抽篮子 (Autodesk Fusion 360 design; units mm, degrees)
part number: 2026-05-02-11-19-45-194
Autodesk Fusion 360 part; units mm, degrees
(part 1 of 4)
sketch "草图1" plane through (0, 0, 0) normal (0, 0, 1) x (1, 0, 0)
  line L0 (-125, -56.5) -> (125, -56.5)
  line L1 (125, -56.5) -> (125, 56.5)
  line L2 (125, 56.5) -> (-125, 56.5)
  line L3 (-125, 56.5) -> (-125, -56.5)
  point P0 (0, -56.5)
  point P1 (-125, 0)
  dimension "d13" = 250
  dimension "d14" = 113
  constraint horizontal L0
  constraint horizontal L2
  constraint vertical L3
  constraint vertical L1
  constraint midpoint L0 P0
  constraint midpoint L3 P1
  constraint vertical origin P0
  constraint horizontal origin P1
  measures "d13" horizontal distance of L0.start L0.end
  measures "d14" vertical distance of L0.start L2.end
extrude "拉伸1" add sketch "草图1" along normal blind 90
fillet "fillet_right_corners" radius 10 2 edges at (125, 56.5, 45) (125, -56.5, 45)
shell "shell_basket" thickness 2 removed faces 1 at (-45, 18.8333, 90)
sketch "草图16" plane through (125, 0, 0) normal (1, 0, 0) x (0, 1, 0)
  line L0 (-46.5, 90) -> (-46.5, 0)
  line L1 (-46.5, 0) -> (46.5, 0)
  line L2 (46.5, 0) -> (46.5, 90)
  line L3 (46.5, 90) -> (-46.5, 90)
  arc A0 (29, 60) -> (29, 82) centre (29, 71) ccw
  arc A1 (-29, 82) -> (-29, 60) centre (-29, 71) ccw
  line L4 (-29, 60) -> (29, 60)
  line L5 (29, 82) -> (-29, 82)
  dimension "d60" = 29
  dimension "d61" = 29
  dimension "d62" = 71
  dimension "d63" = 11
  dimension "d64" = 11
  constraint horizontal L4
  constraint horizontal L5
  constraint horizontal A0.centre A1.centre
  measures "d60" horizontal distance of origin A1.centre
  measures "d61" horizontal distance of origin A0.centre
  measures "d62" vertical distance of origin A1.centre
  measures "d63" radius of A1
  measures "d64" radius of A0
extrude "拉伸16" cut sketch "草图16" against normal blind 3 contours A0 A1 L4 L5
sketch "草图29" plane through (-125, 0, 0) normal (-1, 0, 0) x (0, -1, 0)
  line L0 (-56.5, 0) -> (56.5, 0)
  line L1 (56.5, 0) -> (56.5, 90)
  line L2 (56.5, 90) -> (-56.5, 90)
  line L3 (-56.5, 90) -> (-56.5, 0)
  line L4 (-47.5, 14) -> (-51.8301, 11.5)
  line L5 (-51.8301, 11.5) -> (-51.8301, 6.5)
  line L6 (-51.8301, 6.5) -> (-47.5, 4)
  line L7 (-47.5, 4) -> (-43.1699, 6.5)
  line L8 (-43.1699, 6.5) -> (-43.1699, 11.5)
  line L9 (-43.1699, 11.5) -> (-47.5, 14)
  line L10 (-36.8397, 14) -> (-41.1699, 11.5)
  line L11 (-41.1699, 11.5) -> (-41.1699, 6.5)
  line L12 (-41.1699, 6.5) -> (-36.8397, 4)
  line L13 (-36.8397, 4) -> (-32.5096, 6.5)
  line L14 (-32.5096, 6.5) -> (-32.5096, 11.5)
  line L15 (-32.5096, 11.5) -> (-36.8397, 14)
  line L16 (-26.1795, 14) -> (-30.5096, 11.5)
  line L17 (-30.5096, 11.5) -> (-30.5096, 6.5)
  line L18 (-30.5096, 6.5) -> (-26.1795, 4)
  line L19 (-26.1795, 4) -> (-21.8494, 6.5)
  line L20 (-21.8494, 6.5) -> (-21.8494, 11.5)
  line L21 (-21.8494, 11.5) -> (-26.1795, 14)
  line L22 (-15.5192, 14) -> (-19.8494, 11.5)
  line L23 (-19.8494, 11.5) -> (-19.8494, 6.5)
  line L24 (-19.8494, 6.5) -> (-15.5192, 4)
  line L25 (-15.5192, 4) -> (-11.1891, 6.5)
  line L26 (-11.1891, 6.5) -> (-11.1891, 11.5)
  line L27 (-11.1891, 11.5) -> (-15.5192, 14)
  line L28 (-4.859, 14) -> (-9.1891, 11.5)
  line L29 (-9.1891, 11.5) -> (-9.1891, 6.5)
  line L30 (-9.1891, 6.5) -> (-4.859, 4)
  line L31 (-4.859, 4) -> (-0.5289, 6.5)
  line L32 (-0.5289, 6.5) -> (-0.5289, 11.5)
  line L33 (-0.5289, 11.5) -> (-4.859, 14)
  line L34 (5.8013, 14) -> (1.4711, 11.5)
  line L35 (1.4711, 11.5) -> (1.4711, 6.5)
  line L36 (1.4711, 6.5) -> (5.8013, 4)
  line L37 (5.8013, 4) -> (10.1314, 6.5)
  line L38 (10.1314, 6.5) -> (10.1314, 11.5)
  line L39 (10.1314, 11.5) -> (5.8013, 14)
  line L40 (16.4615, 14) -> (12.1314, 11.5)
  line L41 (12.1314, 11.5) -> (12.1314, 6.5)
  line L42 (12.1314, 6.5) -> (16.4615, 4)
  line L43 (16.4615, 4) -> (20.7917, 6.5)
  line L44 (20.7917, 6.5) -> (20.7917, 11.5)
  line L45 (20.7917, 11.5) -> (16.4615, 14)
  line L46 (27.1218, 14) -> (22.7917, 11.5)
  line L47 (22.7917, 11.5) -> (22.7917, 6.5)
  line L48 (22.7917, 6.5) -> (27.1218, 4)
  line L49 (27.1218, 4) -> (31.4519, 6.5)
  line L50 (31.4519, 6.5) -> (31.4519, 11.5)
  line L51 (31.4519, 11.5) -> (27.1218, 14)
  line L52 (37.782, 14) -> (33.4519, 11.5)
  line L53 (33.4519, 11.5) -> (33.4519, 6.5)
  line L54 (33.4519, 6.5) -> (37.782, 4)
  line L55 (37.782, 4) -> (42.1122, 6.5)
  line L56 (42.1122, 6.5) -> (42.1122, 11.5)
  line L57 (42.1122, 11.5) -> (37.782, 14)
  line L58 (-42.1699, 23.2321) -> (-46.5, 20.7321)
  line L59 (-46.5, 20.7321) -> (-46.5, 15.7321)
  line L60 (-46.5, 15.7321) -> (-42.1699, 13.2321)
  line L61 (-42.1699, 13.2321) -> (-37.8397, 15.7321)
  line L62 (-37.8397, 15.7321) -> (-37.8397, 20.7321)
  line L63 (-37.8397, 20.7321) -> (-42.1699, 23.2321)
  line L64 (-31.5096, 23.2321) -> (-35.8397, 20.7321)
  line L65 (-35.8397, 20.7321) -> (-35.8397, 15.7321)
  line L66 (-35.8397, 15.7321) -> (-31.5096, 13.2321)
  line L67 (-31.5096, 13.2321) -> (-27.1795, 15.7321)
  line L68 (-27.1795, 15.7321) -> (-27.1795, 20.7321)
  line L69 (-27.1795, 20.7321) -> (-31.5096, 23.2321)
  line L70 (-20.8494, 23.2321) -> (-25.1795, 20.7321)
  line L71 (-25.1795, 20.7321) -> (-25.1795, 15.7321)
  line L72 (-25.1795, 15.7321) -> (-20.8494, 13.2321)
  line L73 (-20.8494, 13.2321) -> (-16.5192, 15.7321)
  line L74 (-16.5192, 15.7321) -> (-16.5192, 20.7321)
  line L75 (-16.5192, 20.7321) -> (-20.8494, 23.2321)
  line L76 (-10.1891, 23.2321) -> (-14.5192, 20.7321)
  line L77 (-14.5192, 20.7321) -> (-14.5192, 15.7321)
  line L78 (-14.5192, 15.7321) -> (-10.1891, 13.2321)
  line L79 (-10.1891, 13.2321) -> (-5.859, 15.7321)
  line L80 (-5.859, 15.7321) -> (-5.859, 20.7321)
  line L81 (-5.859, 20.7321) -> (-10.1891, 23.2321)
  line L82 (0.4711, 23.2321) -> (-3.859, 20.7321)
  line L83 (-3.859, 20.7321) -> (-3.859, 15.7321)
  line L84 (-3.859, 15.7321) -> (0.4711, 13.2321)
  line L85 (0.4711, 13.2321) -> (4.8013, 15.7321)
  line L86 (4.8013, 15.7321) -> (4.8013, 20.7321)
  line L87 (4.8013, 20.7321) -> (0.4711, 23.2321)
  line L88 (11.1314, 23.2321) -> (6.8013, 20.7321)
  line L89 (6.8013, 20.7321) -> (6.8013, 15.7321)
  line L90 (6.8013, 15.7321) -> (11.1314, 13.2321)
  line L91 (11.1314, 13.2321) -> (15.4615, 15.7321)
  line L92 (15.4615, 15.7321) -> (15.4615, 20.7321)
  line L93 (15.4615, 20.7321) -> (11.1314, 23.2321)
  line L94 (21.7917, 23.2321) -> (17.4615, 20.7321)
  line L95 (17.4615, 20.7321) -> (17.4615, 15.7321)
  line L96 (17.4615, 15.7321) -> (21.7917, 13.2321)
  line L97 (21.7917, 13.2321) -> (26.1218, 15.7321)
  line L98 (26.1218, 15.7321) -> (26.1218, 20.7321)
  line L99 (26.1218, 20.7321) -> (21.7917, 23.2321)
  line L100 (32.4519, 23.2321) -> (28.1218, 20.7321)
  line L101 (28.1218, 20.7321) -> (28.1218, 15.7321)
  line L102 (28.1218, 15.7321) -> (32.4519, 13.2321)
  line L103 (32.4519, 13.2321) -> (36.782, 15.7321)
  line L104 (36.782, 15.7321) -> (36.782, 20.7321)
  line L105 (36.782, 20.7321) -> (32.4519, 23.2321)
  line L106 (43.1122, 23.2321) -> (38.782, 20.7321)
  line L107 (38.782, 20.7321) -> (38.782, 15.7321)
  line L108 (38.782, 15.7321) -> (43.1122, 13.2321)
  line L109 (43.1122, 13.2321) -> (47.4423, 15.7321)
  line L110 (47.4423, 15.7321) -> (47.4423, 20.7321)
  line L111 (47.4423, 20.7321) -> (43.1122, 23.2321)
  line L112 (-47.5, 32.4641) -> (-51.8301, 29.9641)
  line L113 (-51.8301, 29.9641) -> (-51.8301, 24.9641)
  line L114 (-51.8301, 24.9641) -> (-47.5, 22.4641)
  line L115 (-47.5, 22.4641) -> (-43.1699, 24.9641)
  line L116 (-43.1699, 24.9641) -> (-43.1699, 29.9641)
  line L117 (-43.1699, 29.9641) -> (-47.5, 32.4641)
  line L118 (-36.8397, 32.4641) -> (-41.1699, 29.9641)
  line L119 (-41.1699, 29.9641) -> (-41.1699, 24.9641)
  line L120 (-41.1699, 24.9641) -> (-36.8397, 22.4641)
  line L121 (-36.8397, 22.4641) -> (-32.5096, 24.9641)
  line L122 (-32.5096, 24.9641) -> (-32.5096, 29.9641)
  line L123 (-32.5096, 29.9641) -> (-36.8397, 32.4641)
  line L124 (-26.1795, 32.4641) -> (-30.5096, 29.9641)
  line L125 (-30.5096, 29.9641) -> (-30.5096, 24.9641)
  line L126 (-30.5096, 24.9641) -> (-26.1795, 22.4641)
  line L127 (-26.1795, 22.4641) -> (-21.8494, 24.9641)
  line L128 (-21.8494, 24.9641) -> (-21.8494, 29.9641)
  line L129 (-21.8494, 29.9641) -> (-26.1795, 32.4641)
  line L130 (-15.5192, 32.4641) -> (-19.8494, 29.9641)
  line L131 (-19.8494, 29.9641) -> (-19.8494, 24.9641)
  line L132 (-19.8494, 24.9641) -> (-15.5192, 22.4641)
  line L133 (-15.5192, 22.4641) -> (-11.1891, 24.9641)
  line L134 (-11.1891, 24.9641) -> (-11.1891, 29.9641)
  line L135 (-11.1891, 29.9641) -> (-15.5192, 32.4641)
  line L136 (-4.859, 32.4641) -> (-9.1891, 29.9641)
  line L137 (-9.1891, 29.9641) -> (-9.1891, 24.9641)
  line L138 (-9.1891, 24.9641) -> (-4.859, 22.4641)
  line L139 (-4.859, 22.4641) -> (-0.5289, 24.9641)
  line L140 (-0.5289, 24.9641) -> (-0.5289, 29.9641)
  line L141 (-0.5289, 29.9641) -> (-4.859, 32.4641)
  line L142 (5.8013, 32.4641) -> (1.4711, 29.9641)
  line L143 (1.4711, 29.9641) -> (1.4711, 24.9641)
  line L144 (1.4711, 24.9641) -> (5.8013, 22.4641)
  line L145 (5.8013, 22.4641) -> (10.1314, 24.9641)
  line L146 (10.1314, 24.9641) -> (10.1314, 29.9641)
  line L147 (10.1314, 29.9641) -> (5.8013, 32.4641)
  line L148 (16.4615, 32.4641) -> (12.1314, 29.9641)
  line L149 (12.1314, 29.9641) -> (12.1314, 24.9641)
  line L150 (12.1314, 24.9641) -> (16.4615, 22.4641)
  line L151 (16.4615, 22.4641) -> (20.7917, 24.9641)
  line L152 (20.7917, 24.9641) -> (20.7917, 29.9641)
  line L153 (20.7917, 29.9641) -> (16.4615, 32.4641)
  line L154 (27.1218, 32.4641) -> (22.7917, 29.9641)
  line L155 (22.7917, 29.9641) -> (22.7917, 24.9641)
  line L156 (22.7917, 24.9641) -> (27.1218, 22.4641)
  line L157 (27.1218, 22.4641) -> (31.4519, 24.9641)
  line L158 (31.4519, 24.9641) -> (31.4519, 29.9641)
  line L159 (31.4519, 29.9641) -> (27.1218, 32.4641)
  line L160 (37.782, 32.4641) -> (33.4519, 29.9641)
  line L161 (33.4519, 29.9641) -> (33.4519, 24.9641)
  line L162 (33.4519, 24.9641) -> (37.782, 22.4641)
  line L163 (37.782, 22.4641) -> (42.1122, 24.9641)
  line L164 (42.1122, 24.9641) -> (42.1122, 29.9641)
  line L165 (42.1122, 29.9641) -> (37.782, 32.4641)
  line L166 (-42.1699, 41.6962) -> (-46.5, 39.1962)
  line L167 (-46.5, 39.1962) -> (-46.5, 34.1962)
  line L168 (-46.5, 34.1962) -> (-42.1699, 31.6962)
  line L169 (-42.1699, 31.6962) -> (-37.8397, 34.1962)
  line L170 (-37.8397, 34.1962) -> (-37.8397, 39.1962)
  line L171 (-37.8397, 39.1962) -> (-42.1699, 41.6962)
  line L172 (-31.5096, 41.6962) -> (-35.8397, 39.1962)
  line L173 (-35.8397, 39.1962) -> (-35.8397, 34.1962)
  line L174 (-35.8397, 34.1962) -> (-31.5096, 31.6962)
  line L175 (-31.5096, 31.6962) -> (-27.1795, 34.1962)
  line L176 (-27.1795, 34.1962) -> (-27.1795, 39.1962)
  line L177 (-27.1795, 39.1962) -> (-31.5096, 41.6962)
  line L178 (-20.8494, 41.6962) -> (-25.1795, 39.1962)
  line L179 (-25.1795, 39.1962) -> (-25.1795, 34.1962)
  line L180 (-25.1795, 34.1962) -> (-20.8494, 31.6962)
  line L181 (-20.8494, 31.6962) -> (-16.5192, 34.1962)
  line L182 (-16.5192, 34.1962) -> (-16.5192, 39.1962)
  line L183 (-16.5192, 39.1962) -> (-20.8494, 41.6962)
  line L184 (-10.1891, 41.6962) -> (-14.5192, 39.1962)
  line L185 (-14.5192, 39.1962) -> (-14.5192, 34.1962)
  line L186 (-14.5192, 34.1962) -> (-10.1891, 31.6962)
  line L187 (-10.1891, 31.6962) -> (-5.859, 34.1962)
  line L188 (-5.859, 34.1962) -> (-5.859, 39.1962)
  line L189 (-5.859, 39.1962) -> (-10.1891, 41.6962)
  line L190 (0.4711, 41.6962) -> (-3.859, 39.1962)
  line L191 (-3.859, 39.1962) -> (-3.859, 34.1962)
  line L192 (-3.859, 34.1962) -> (0.4711, 31.6962)
  line L193 (0.4711, 31.6962) -> (4.8013, 34.1962)
  line L194 (4.8013, 34.1962) -> (4.8013, 39.1962)
  line L195 (4.8013, 39.1962) -> (0.4711, 41.6962)
  line L196 (11.1314, 41.6962) -> (6.8013, 39.1962)
  line L197 (6.8013, 39.1962) -> (6.8013, 34.1962)
  line L198 (6.8013, 34.1962) -> (11.1314, 31.6962)
  line L199 (11.1314, 31.6962) -> (15.4615, 34.1962)
  line L200 (15.4615, 34.1962) -> (15.4615, 39.1962)
  line L201 (15.4615, 39.1962) -> (11.1314, 41.6962)
  line L202 (21.7917, 41.6962) -> (17.4615, 39.1962)
  line L203 (17.4615, 39.1962) -> (17.4615, 34.1962)
  line L204 (17.4615, 34.1962) -> (21.7917, 31.6962)
  line L205 (21.7917, 31.6962) -> (26.1218, 34.1962)
  line L206 (26.1218, 34.1962) -> (26.1218, 39.1962)
  line L207 (26.1218, 39.1962) -> (21.7917, 41.6962)
  line L208 (32.4519, 41.6962) -> (28.1218, 39.1962)
  line L209 (28.1218, 39.1962) -> (28.1218, 34.1962)
  line L210 (28.1218, 34.1962) -> (32.4519, 31.6962)
  line L211 (32.4519, 31.6962) -> (36.782, 34.1962)
  line L212 (36.782, 34.1962) -> (36.782, 39.1962)
  line L213 (36.782, 39.1962) -> (32.4519, 41.6962)
  line L214 (43.1122, 41.6962) -> (38.782, 39.1962)
  line L215 (38.782, 39.1962) -> (38.782, 34.1962)
  line L216 (38.782, 34.1962) -> (43.1122, 31.6962)
  line L217 (43.1122, 31.6962) -> (47.4423, 34.1962)
  line L218 (47.4423, 34.1962) -> (47.4423, 39.1962)
  line L219 (47.4423, 39.1962) -> (43.1122, 41.6962)
  line L220 (-47.5, 50.9282) -> (-51.8301, 48.4282)
  line L221 (-51.8301, 48.4282) -> (-51.8301, 43.4282)
  line L222 (-51.8301, 43.4282) -> (-47.5, 40.9282)
  line L223 (-47.5, 40.9282) -> (-43.1699, 43.4282)
  line L224 (-43.1699, 43.4282) -> (-43.1699, 48.4282)
  line L225 (-43.1699, 48.4282) -> (-47.5, 50.9282)
  line L226 (-36.8397, 50.9282) -> (-41.1699, 48.4282)
  line L227 (-41.1699, 48.4282) -> (-41.1699, 43.4282)
  line L228 (-41.1699, 43.4282) -> (-36.8397, 40.9282)
  line L229 (-36.8397, 40.9282) -> (-32.5096, 43.4282)
  line L230 (-32.5096, 43.4282) -> (-32.5096, 48.4282)
  line L231 (-32.5096, 48.4282) -> (-36.8397, 50.9282)
  line L232 (-26.1795, 50.9282) -> (-30.5096, 48.4282)
  line L233 (-30.5096, 48.4282) -> (-30.5096, 43.4282)
  line L234 (-30.5096, 43.4282) -> (-26.1795, 40.9282)
  line L235 (-26.1795, 40.9282) -> (-21.8494, 43.4282)
  line L236 (-21.8494, 43.4282) -> (-21.8494, 48.4282)
  line L237 (-21.8494, 48.4282) -> (-26.1795, 50.9282)
  line L238 (-15.5192, 50.9282) -> (-19.8494, 48.4282)
  line L239 (-19.8494, 48.4282) -> (-19.8494, 43.4282)
  line L240 (-19.8494, 43.4282) -> (-15.5192, 40.9282)
  line L241 (-15.5192, 40.9282) -> (-11.1891, 43.4282)
  line L242 (-11.1891, 43.4282) -> (-11.1891, 48.4282)
  line L243 (-11.1891, 48.4282) -> (-15.5192, 50.9282)
  line L244 (-4.859, 50.9282) -> (-9.1891, 48.4282)
  line L245 (-9.1891, 48.4282) -> (-9.1891, 43.4282)
  line L246 (-9.1891, 43.4282) -> (-4.859, 40.9282)
  line L247 (-4.859, 40.9282) -> (-0.5289, 43.4282)
  line L248 (-0.5289, 43.4282) -> (-0.5289, 48.4282)
  line L249 (-0.5289, 48.4282) -> (-4.859, 50.9282)
  line L250 (5.8013, 50.9282) -> (1.4711, 48.4282)
  line L251 (1.4711, 48.4282) -> (1.4711, 43.4282)
  line L252 (1.4711, 43.4282) -> (5.8013, 40.9282)
  line L253 (5.8013, 40.9282) -> (10.1314, 43.4282)
  line L254 (10.1314, 43.4282) -> (10.1314, 48.4282)
  line L255 (10.1314, 48.4282) -> (5.8013, 50.9282)
  line L256 (16.4615, 50.9282) -> (12.1314, 48.4282)
  line L257 (12.1314, 48.4282) -> (12.1314, 43.4282)
  line L258 (12.1314, 43.4282) -> (16.4615, 40.9282)
  line L259 (16.4615, 40.9282) -> (20.7917, 43.4282)
  line L260 (20.7917, 43.4282) -> (20.7917, 48.4282)
  line L261 (20.7917, 48.4282) -> (16.4615, 50.9282)
  line L262 (27.1218, 50.9282) -> (22.7917, 48.4282)
  line L263 (22.7917, 48.4282) -> (22.7917, 43.4282)
  line L264 (22.7917, 43.4282) -> (27.1218, 40.9282)
  line L265 (27.1218, 40.9282) -> (31.4519, 43.4282)
  line L266 (31.4519, 43.4282) -> (31.4519, 48.4282)
  line L267 (31.4519, 48.4282) -> (27.1218, 50.9282)
  line L268 (37.782, 50.9282) -> (33.4519, 48.4282)
  line L269 (33.4519, 48.4282) -> (33.4519, 43.4282)
  line L270 (33.4519, 43.4282) -> (37.782, 40.9282)
  line L271 (37.782, 40.9282) -> (42.1122, 43.4282)
  line L272 (42.1122, 43.4282) -> (42.1122, 48.4282)
  line L273 (42.1122, 48.4282) -> (37.782, 50.9282)
  line L274 (-42.1699, 60.1603) -> (-46.5, 57.6603)
  line L275 (-46.5, 57.6603) -> (-46.5, 52.6603)
  line L276 (-46.5, 52.6603) -> (-42.1699, 50.1603)
  line L277 (-42.1699, 50.1603) -> (-37.8397, 52.6603)
  line L278 (-37.8397, 52.6603) -> (-37.8397, 57.6603)
  line L279 (-37.8397, 57.6603) -> (-42.1699, 60.1603)
  line L280 (-31.5096, 60.1603) -> (-35.8397, 57.6603)
  line L281 (-35.8397, 57.6603) -> (-35.8397, 52.6603)
  line L282 (-35.8397, 52.6603) -> (-31.5096, 50.1603)
  line L283 (-31.5096, 50.1603) -> (-27.1795, 52.6603)
  line L284 (-27.1795, 52.6603) -> (-27.1795, 57.6603)
  line L285 (-27.1795, 57.6603) -> (-31.5096, 60.1603)
  line L286 (-20.8494, 60.1603) -> (-25.1795, 57.6603)
  line L287 (-25.1795, 57.6603) -> (-25.1795, 52.6603)
  line L288 (-25.1795, 52.6603) -> (-20.8494, 50.1603)
  line L289 (-20.8494, 50.1603) -> (-16.5192, 52.6603)
  line L290 (-16.5192, 52.6603) -> (-16.5192, 57.6603)
  line L291 (-16.5192, 57.6603) -> (-20.8494, 60.1603)
  line L292 (-10.1891, 60.1603) -> (-14.5192, 57.6603)
  line L293 (-14.5192, 57.6603) -> (-14.5192, 52.6603)
  line L294 (-14.5192, 52.6603) -> (-10.1891, 50.1603)
  line L295 (-10.1891, 50.1603) -> (-5.859, 52.6603)
  line L296 (-5.859, 52.6603) -> (-5.859, 57.6603)
  line L297 (-5.859, 57.6603) -> (-10.1891, 60.1603)
  line L298 (0.4711, 60.1603) -> (-3.859, 57.6603)
  line L299 (-3.859, 57.6603) -> (-3.859, 52.6603)
  line L300 (-3.859, 52.6603) -> (0.4711, 50.1603)
  line L301 (0.4711, 50.1603) -> (4.8013, 52.6603)
  line L302 (4.8013, 52.6603) -> (4.8013, 57.6603)
  line L303 (4.8013, 57.6603) -> (0.4711, 60.1603)
  line L304 (11.1314, 60.1603) -> (6.8013, 57.6603)
  line L305 (6.8013, 57.6603) -> (6.8013, 52.6603)
  line L306 (6.8013, 52.6603) -> (11.1314, 50.1603)
  line L307 (11.1314, 50.1603) -> (15.4615, 52.6603)
  line L308 (15.4615, 52.6603) -> (15.4615, 57.6603)
  line L309 (15.4615, 57.6603) -> (11.1314, 60.1603)
  line L310 (21.7917, 60.1603) -> (17.4615, 57.6603)
  line L311 (17.4615, 57.6603) -> (17.4615, 52.6603)
  line L312 (17.4615, 52.6603) -> (21.7917, 50.1603)
  line L313 (21.7917, 50.1603) -> (26.1218, 52.6603)
  line L314 (26.1218, 52.6603) -> (26.1218, 57.6603)
  line L315 (26.1218, 57.6603) -> (21.7917, 60.1603)
  line L316 (32.4519, 60.1603) -> (28.1218, 57.6603)
  line L317 (28.1218, 57.6603) -> (28.1218, 52.6603)
  line L318 (28.1218, 52.6603) -> (32.4519, 50.1603)
  line L319 (32.4519, 50.1603) -> (36.782, 52.6603)
  line L320 (36.782, 52.6603) -> (36.782, 57.6603)
  line L321 (36.782, 57.6603) -> (32.4519, 60.1603)
  line L322 (43.1122, 60.1603) -> (38.782, 57.6603)
  line L323 (38.782, 57.6603) -> (38.782, 52.6603)
  line L324 (38.782, 52.6603) -> (43.1122, 50.1603)
  line L325 (43.1122, 50.1603) -> (47.4423, 52.6603)
  line L326 (47.4423, 52.6603) -> (47.4423, 57.6603)
  line L327 (47.4423, 57.6603) -> (43.1122, 60.1603)
  line L328 (-47.5, 69.3923) -> (-51.8301, 66.8923)
  line L329 (-51.8301, 66.8923) -> (-51.8301, 61.8923)
  line L330 (-51.8301, 61.8923) -> (-47.5, 59.3923)
  line L331 (-47.5, 59.3923) -> (-43.1699, 61.8923)
  line L332 (-43.1699, 61.8923) -> (-43.1699, 66.8923)
  line L333 (-43.1699, 66.8923) -> (-47.5, 69.3923)
  line L334 (-36.8397, 69.3923) -> (-41.1699, 66.8923)
  line L335 (-41.1699, 66.8923) -> (-41.1699, 61.8923)
  line L336 (-41.1699, 61.8923) -> (-36.8397, 59.3923)
  line L337 (-36.8397, 59.3923) -> (-32.5096, 61.8923)
  line L338 (-32.5096, 61.8923) -> (-32.5096, 66.8923)
  line L339 (-32.5096, 66.8923) -> (-36.8397, 69.3923)
  line L340 (-26.1795, 69.3923) -> (-30.5096, 66.8923)
  line L341 (-30.5096, 66.8923) -> (-30.5096, 61.8923)
  line L342 (-30.5096, 61.8923) -> (-26.1795, 59.3923)
  line L343 (-26.1795, 59.3923) -> (-21.8494, 61.8923)
  line L344 (-21.8494, 61.8923) -> (-21.8494, 66.8923)
  line L345 (-21.8494, 66.8923) -> (-26.1795, 69.3923)
  line L346 (-15.5192, 69.3923) -> (-19.8494, 66.8923)
  line L347 (-19.8494, 66.8923) -> (-19.8494, 61.8923)
  line L348 (-19.8494, 61.8923) -> (-15.5192, 59.3923)
  line L349 (-15.5192, 59.3923) -> (-11.1891, 61.8923)
  line L350 (-11.1891, 61.8923) -> (-11.1891, 66.8923)
  line L351 (-11.1891, 66.8923) -> (-15.5192, 69.3923)
  line L352 (-4.859, 69.3923) -> (-9.1891, 66.8923)
  line L353 (-9.1891, 66.8923) -> (-9.1891, 61.8923)
  line L354 (-9.1891, 61.8923) -> (-4.859, 59.3923)
  line L355 (-4.859, 59.3923) -> (-0.5289, 61.8923)
  line L356 (-0.5289, 61.8923) -> (-0.5289, 66.8923)
  line L357 (-0.5289, 66.8923) -> (-4.859, 69.3923)
  line L358 (5.8013, 69.3923) -> (1.4711, 66.8923)
  line L359 (1.4711, 66.8923) -> (1.4711, 61.8923)
  line L360 (1.4711, 61.8923) -> (5.8013, 59.3923)
  line L361 (5.8013, 59.3923) -> (10.1314, 61.8923)
  line L362 (10.1314, 61.8923) -> (10.1314, 66.8923)
  line L363 (10.1314, 66.8923) -> (5.8013, 69.3923)
  line L364 (16.4615, 69.3923) -> (12.1314, 66.8923)
  line L365 (12.1314, 66.8923) -> (12.1314, 61.8923)
  line L366 (12.1314, 61.8923) -> (16.4615, 59.3923)
  line L367 (16.4615, 59.3923) -> (20.7917, 61.8923)
  line L368 (20.7917, 61.8923) -> (20.7917, 66.8923)
  line L369 (20.7917, 66.8923) -> (16.4615, 69.3923)
  line L370 (27.1218, 69.3923) -> (22.7917, 66.8923)
  line L371 (22.7917, 66.8923) -> (22.7917, 61.8923)
  line L372 (22.7917, 61.8923) -> (27.1218, 59.3923)
  line L373 (27.1218, 59.3923) -> (31.4519, 61.8923)
  line L374 (31.4519, 61.8923) -> (31.4519, 66.8923)
  line L375 (31.4519, 66.8923) -> (27.1218, 69.3923)
  line L376 (37.782, 69.3923) -> (33.4519, 66.8923)
  line L377 (33.4519, 66.8923) -> (33.4519, 61.8923)
  line L378 (33.4519, 61.8923) -> (37.782, 59.3923)
  line L379 (37.782, 59.3923) -> (42.1122, 61.8923)
  line L380 (42.1122, 61.8923) -> (42.1122, 66.8923)
  line L381 (42.1122, 66.8923) -> (37.782, 69.3923)
  line L382 (-42.1699, 78.6244) -> (-46.5, 76.1244)
  line L383 (-46.5, 76.1244) -> (-46.5, 71.1244)
  line L384 (-46.5, 71.1244) -> (-42.1699, 68.6244)
  line L385 (-42.1699, 68.6244) -> (-37.8397, 71.1244)
  line L386 (-37.8397, 71.1244) -> (-37.8397, 76.1244)
  line L387 (-37.8397, 76.1244) -> (-42.1699, 78.6244)
  line L388 (-31.5096, 78.6244) -> (-35.8397, 76.1244)
  line L389 (-35.8397, 76.1244) -> (-35.8397, 71.1244)
  line L390 (-35.8397, 71.1244) -> (-31.5096, 68.6244)
  line L391 (-31.5096, 68.6244) -> (-27.1795, 71.1244)
  line L392 (-27.1795, 71.1244) -> (-27.1795, 76.1244)
  line L393 (-27.1795, 76.1244) -> (-31.5096, 78.6244)
  line L394 (-20.8494, 78.6244) -> (-25.1795, 76.1244)
  line L395 (-25.1795, 76.1244) -> (-25.1795, 71.1244)
  line L396 (-25.1795, 71.1244) -> (-20.8494, 68.6244)
  line L397 (-20.8494, 68.6244) -> (-16.5192, 71.1244)
  line L398 (-16.5192, 71.1244) -> (-16.5192, 76.1244)
  line L399 (-16.5192, 76.1244) -> (-20.8494, 78.6244)
  line L400 (-10.1891, 78.6244) -> (-14.5192, 76.1244)
  line L401 (-14.5192, 76.1244) -> (-14.5192, 71.1244)
  line L402 (-14.5192, 71.1244) -> (-10.1891, 68.6244)
  line L403 (-10.1891, 68.6244) -> (-5.859, 71.1244)
  line L404 (-5.859, 71.1244) -> (-5.859, 76.1244)
  line L405 (-5.859, 76.1244) -> (-10.1891, 78.6244)
  line L406 (0.4711, 78.6244) -> (-3.859, 76.1244)
  line L407 (-3.859, 76.1244) -> (-3.859, 71.1244)
  line L408 (-3.859, 71.1244) -> (0.4711, 68.6244)
  line L409 (0.4711, 68.6244) -> (4.8013, 71.1244)
  line L410 (4.8013, 71.1244) -> (4.8013, 76.1244)
  line L411 (4.8013, 76.1244) -> (0.4711, 78.6244)
  line L412 (11.1314, 78.6244) -> (6.8013, 76.1244)
  line L413 (6.8013, 76.1244) -> (6.8013, 71.1244)
  line L414 (6.8013, 71.1244) -> (11.1314, 68.6244)
  line L415 (11.1314, 68.6244) -> (15.4615, 71.1244)
  line L416 (15.4615, 71.1244) -> (15.4615, 76.1244)
  line L417 (15.4615, 76.1244) -> (11.1314, 78.6244)
  line L418 (21.7917, 78.6244) -> (17.4615, 76.1244)
  line L419 (17.4615, 76.1244) -> (17.4615, 71.1244)
  line L420 (17.4615, 71.1244) -> (21.7917, 68.6244)
  line L421 (21.7917, 68.6244) -> (26.1218, 71.1244)
  line L422 (26.1218, 71.1244) -> (26.1218, 76.1244)
  line L423 (26.1218, 76.1244) -> (21.7917, 78.6244)
  line L424 (32.4519, 78.6244) -> (28.1218, 76.1244)
  line L425 (28.1218, 76.1244) -> (28.1218, 71.1244)
  line L426 (28.1218, 71.1244) -> (32.4519, 68.6244)
  line L427 (32.4519, 68.6244) -> (36.782, 71.1244)
  line L428 (36.782, 71.1244) -> (36.782, 76.1244)
  line L429 (36.782, 76.1244) -> (32.4519, 78.6244)
  line L430 (43.1122, 78.6244) -> (38.782, 76.1244)
  line L431 (38.782, 76.1244) -> (38.782, 71.1244)
  line L432 (38.782, 71.1244) -> (43.1122, 68.6244)
  line L433 (43.1122, 68.6244) -> (47.4423, 71.1244)
  line L434 (47.4423, 71.1244) -> (47.4423, 76.1244)
  line L435 (47.4423, 76.1244) -> (43.1122, 78.6244)
extrude "拉伸29" cut sketch "草图29" against normal blind 3 contours L4 L5 L6 L7 L8 L9 | L10 L11 L12 L13 L14 L15 | L16 L17 L18 L19 L20 L21 | L22 L23 L24 L25 L26 L27 | L28 L29 L30 L31 L32 L33 | L34 L35 L36 L37 L38 L39 | L40 L41 L42 L43 L44 L45 | L46 L47 L48 L49 L50 L51 | L52 L53 L54 L55 L56 L57 | L58 L59 L60 L61 L62 L63 | L64 L65 L66 L67 L68 L69 | L70 L71 L72 L73 L74 L75 | L76 L77 L78 L79 L80 L81 | L82 L83 L84 L85 L86 L87 | L88 L89 L90 L91 L92 L93 | L94 L95 L96 L97 L98 L99 | L100 L101 L102 L103 L104 L105 | L106 L107 L108 L109 L110 L111 | L112 L113 L114 L115 L116 L117 | L118 L119 L120 L121 L122 L123 | L124 L125 L126 L127 L128 L129 | L130 L131 L132 L133 L134 L135 | L136 L137 L138 L139 L140 L141 | L142 L143 L144 L145 L146 L147 | L148 L149 L150 L151 L152 L153 | L154 L155 L156 L157 L158 L159 | L160 L161 L162 L163 L164 L165 | L166 L167 L168 L169 L170 L171 | L172 L173 L174 L175 L176 L177 | L178 L179 L180 L181 L182 L183 | L184 L185 L186 L187 L188 L189 | L190 L191 L192 L193 L194 L195 | L196 L197 L198 L199 L200 L201 | L202 L203 L204 L205 L206 L207 | L208 L209 L210 L211 L212 L213 | L214 L215 L216 L217 L218 L219 | L220 L221 L222 L223 L224 L225 | L226 L227 L228 L229 L230 L231 | L232 L233 L234 L235 L236 L237 | L238 L239 L240 L241 L242 L243 | L244 L245 L246 L247 L248 L249 | L250 L251 L252 L253 L254 L255 | L256 L257 L258 L259 L260 L261 | L262 L263 L264 L265 L266 L267 | L268 L269 L270 L271 L272 L273 | L274 L275 L276 L277 L278 L279 | L280 L281 L282 L283 L284 L285 | L286 L287 L288 L289 L290 L291 | L292 L293 L294 L295 L296 L297 | L298 L299 L300 L301 L302 L303 | L304 L305 L306 L307 L308 L309 | L310 L311 L312 L313 L314 L315 | L316 L317 L318 L319 L320 L321 | L322 L323 L324 L325 L326 L327 | L328 L329 L330 L331 L332 L333 | L334 L335 L336 L337 L338 L339 | L340 L341 L342 L343 L344 L345 | L346 L347 L348 L349 L350 L351 | L352 L353 L354 L355 L356 L357 | L358 L359 L360 L361 L362 L363 | L364 L365 L366 L367 L368 L369 | L370 L371 L372 L373 L374 L375 | L376 L377 L378 L379 L380 L381 | L382 L383 L384 L385 L386 L387 | L388 L389 L390 L391 L392 L393 | L394 L395 L396 L397 L398 L399 | L400 L401 L402 L403 L404 L405 | L406 L407 L408 L409 L410 L411 | L412 L413 L414 L415 L416 L417 | L418 L419 L420 L421 L422 L423 | L424 L425 L426 L427 L428 L429 | L430 L431 L432 L433 L434 L435
sketch "草图30" plane through (0, -56.5, 0) normal (0, -1, 0) x (1, 0, 0)
  line L0 (115, 0) -> (115, 90)
  line L1 (115, 90) -> (-125, 90)
  line L2 (-125, 90) -> (-125, 0)
  line L3 (-125, 0) -> (115, 0)
  line L4 (-116, 14) -> (-120.3301, 11.5)
  line L5 (-120.3301, 11.5) -> (-120.3301, 6.5)
  line L6 (-120.3301, 6.5) -> (-116, 4)
  line L7 (-116, 4) -> (-111.6699, 6.5)
  line L8 (-111.6699, 6.5) -> (-111.6699, 11.5)
  line L9 (-111.6699, 11.5) -> (-116, 14)
  line L10 (-105.3397, 14) -> (-109.6699, 11.5)
  line L11 (-109.6699, 11.5) -> (-109.6699, 6.5)
  line L12 (-109.6699, 6.5) -> (-105.3397, 4)
  line L13 (-105.3397, 4) -> (-101.0096, 6.5)
  line L14 (-101.0096, 6.5) -> (-101.0096, 11.5)
  line L15 (-101.0096, 11.5) -> (-105.3397, 14)
  line L16 (-94.6795, 14) -> (-99.0096, 11.5)
  line L17 (-99.0096, 11.5) -> (-99.0096, 6.5)
  line L18 (-99.0096, 6.5) -> (-94.6795, 4)
  line L19 (-94.6795, 4) -> (-90.3494, 6.5)
  line L20 (-90.3494, 6.5) -> (-90.3494, 11.5)
  line L21 (-90.3494, 11.5) -> (-94.6795, 14)
  line L22 (-84.0192, 14) -> (-88.3494, 11.5)
  line L23 (-88.3494, 11.5) -> (-88.3494, 6.5)
  line L24 (-88.3494, 6.5) -> (-84.0192, 4)
  line L25 (-84.0192, 4) -> (-79.6891, 6.5)
  line L26 (-79.6891, 6.5) -> (-79.6891, 11.5)
  line L27 (-79.6891, 11.5) -> (-84.0192, 14)
  line L28 (-73.359, 14) -> (-77.6891, 11.5)
  line L29 (-77.6891, 11.5) -> (-77.6891, 6.5)
  line L30 (-77.6891, 6.5) -> (-73.359, 4)
  line L31 (-73.359, 4) -> (-69.0289, 6.5)
  line L32 (-69.0289, 6.5) -> (-69.0289, 11.5)
  line L33 (-69.0289, 11.5) -> (-73.359, 14)
  line L34 (-62.6987, 14) -> (-67.0289, 11.5)
  line L35 (-67.0289, 11.5) -> (-67.0289, 6.5)
  line L36 (-67.0289, 6.5) -> (-62.6987, 4)
  line L37 (-62.6987, 4) -> (-58.3686, 6.5)
  line L38 (-58.3686, 6.5) -> (-58.3686, 11.5)
  line L39 (-58.3686, 11.5) -> (-62.6987, 14)
  line L40 (-52.0385, 14) -> (-56.3686, 11.5)
  line L41 (-56.3686, 11.5) -> (-56.3686, 6.5)
  line L42 (-56.3686, 6.5) -> (-52.0385, 4)
  line L43 (-52.0385, 4) -> (-47.7083, 6.5)
  line L44 (-47.7083, 6.5) -> (-47.7083, 11.5)
  line L45 (-47.7083, 11.5) -> (-52.0385, 14)
  line L46 (-41.3782, 14) -> (-45.7083, 11.5)
  line L47 (-45.7083, 11.5) -> (-45.7083, 6.5)
  line L48 (-45.7083, 6.5) -> (-41.3782, 4)
  line L49 (-41.3782, 4) -> (-37.0481, 6.5)
  line L50 (-37.0481, 6.5) -> (-37.0481, 11.5)
  line L51 (-37.0481, 11.5) -> (-41.3782, 14)
  line L52 (-30.718, 14) -> (-35.0481, 11.5)
  line L53 (-35.0481, 11.5) -> (-35.0481, 6.5)
  line L54 (-35.0481, 6.5) -> (-30.718, 4)
  line L55 (-30.718, 4) -> (-26.3878, 6.5)
  line L56 (-26.3878, 6.5) -> (-26.3878, 11.5)
  line L57 (-26.3878, 11.5) -> (-30.718, 14)
  line L58 (-20.0577, 14) -> (-24.3878, 11.5)
  line L59 (-24.3878, 11.5) -> (-24.3878, 6.5)
  line L60 (-24.3878, 6.5) -> (-20.0577, 4)
  line L61 (-20.0577, 4) -> (-15.7276, 6.5)
  line L62 (-15.7276, 6.5) -> (-15.7276, 11.5)
  line L63 (-15.7276, 11.5) -> (-20.0577, 14)
  line L64 (-9.3975, 14) -> (-13.7276, 11.5)
  line L65 (-13.7276, 11.5) -> (-13.7276, 6.5)
  line L66 (-13.7276, 6.5) -> (-9.3975, 4)
  line L67 (-9.3975, 4) -> (-5.0673, 6.5)
  line L68 (-5.0673, 6.5) -> (-5.0673, 11.5)
  line L69 (-5.0673, 11.5) -> (-9.3975, 14)
  line L70 (1.2628, 14) -> (-3.0673, 11.5)
  line L71 (-3.0673, 11.5) -> (-3.0673, 6.5)
  line L72 (-3.0673, 6.5) -> (1.2628, 4)
  line L73 (1.2628, 4) -> (5.5929, 6.5)
  line L74 (5.5929, 6.5) -> (5.5929, 11.5)
  line L75 (5.5929, 11.5) -> (1.2628, 14)
  line L76 (11.923, 14) -> (7.5929, 11.5)
  line L77 (7.5929, 11.5) -> (7.5929, 6.5)
  line L78 (7.5929, 6.5) -> (11.923, 4)
  line L79 (11.923, 4) -> (16.2532, 6.5)
  line L80 (16.2532, 6.5) -> (16.2532, 11.5)
  line L81 (16.2532, 11.5) -> (11.923, 14)
  line L82 (22.5833, 14) -> (18.2532, 11.5)
  line L83 (18.2532, 11.5) -> (18.2532, 6.5)
  line L84 (18.2532, 6.5) -> (22.5833, 4)
  line L85 (22.5833, 4) -> (26.9134, 6.5)
  line L86 (26.9134, 6.5) -> (26.9134, 11.5)
  line L87 (26.9134, 11.5) -> (22.5833, 14)
  line L88 (33.2436, 14) -> (28.9134, 11.5)
  line L89 (28.9134, 11.5) -> (28.9134, 6.5)
  line L90 (28.9134, 6.5) -> (33.2436, 4)
  line L91 (33.2436, 4) -> (37.5737, 6.5)
  line L92 (37.5737, 6.5) -> (37.5737, 11.5)
  line L93 (37.5737, 11.5) -> (33.2436, 14)
  line L94 (43.9038, 14) -> (39.5737, 11.5)
  line L95 (39.5737, 11.5) -> (39.5737, 6.5)
  line L96 (39.5737, 6.5) -> (43.9038, 4)
  line L97 (43.9038, 4) -> (48.2339, 6.5)
  line L98 (48.2339, 6.5) -> (48.2339, 11.5)
  line L99 (48.2339, 11.5) -> (43.9038, 14)
  line L100 (54.5641, 14) -> (50.2339, 11.5)
  line L101 (50.2339, 11.5) -> (50.2339, 6.5)
  line L102 (50.2339, 6.5) -> (54.5641, 4)
  line L103 (54.5641, 4) -> (58.8942, 6.5)
  line L104 (58.8942, 6.5) -> (58.8942, 11.5)
  line L105 (58.8942, 11.5) -> (54.5641, 14)
  line L106 (65.2243, 14) -> (60.8942, 11.5)
  line L107 (60.8942, 11.5) -> (60.8942, 6.5)
  line L108 (60.8942, 6.5) -> (65.2243, 4)
  line L109 (65.2243, 4) -> (69.5544, 6.5)
  line L110 (69.5544, 6.5) -> (69.5544, 11.5)
  line L111 (69.5544, 11.5) -> (65.2243, 14)
  line L112 (75.8846, 14) -> (71.5544, 11.5)
  line L113 (71.5544, 11.5) -> (71.5544, 6.5)
  line L114 (71.5544, 6.5) -> (75.8846, 4)
  line L115 (75.8846, 4) -> (80.2147, 6.5)
  line L116 (80.2147, 6.5) -> (80.2147, 11.5)
  line L117 (80.2147, 11.5) -> (75.8846, 14)
  line L118 (86.5448, 14) -> (82.2147, 11.5)
  line L119 (82.2147, 11.5) -> (82.2147, 6.5)
  line L120 (82.2147, 6.5) -> (86.5448, 4)
  line L121 (86.5448, 4) -> (90.875, 6.5)
  line L122 (90.875, 6.5) -> (90.875, 11.5)
  line L123 (90.875, 11.5) -> (86.5448, 14)
  line L124 (97.2051, 14) -> (92.875, 11.5)
  line L125 (92.875, 11.5) -> (92.875, 6.5)
  line L126 (92.875, 6.5) -> (97.2051, 4)
  line L127 (97.2051, 4) -> (101.5352, 6.5)
  line L128 (101.5352, 6.5) -> (101.5352, 11.5)
  line L129 (101.5352, 11.5) -> (97.2051, 14)
  line L130 (-110.6699, 23.2321) -> (-115, 20.7321)
  line L131 (-115, 20.7321) -> (-115, 15.7321)
  line L132 (-115, 15.7321) -> (-110.6699, 13.2321)
  line L133 (-110.6699, 13.2321) -> (-106.3397, 15.7321)
  line L134 (-106.3397, 15.7321) -> (-106.3397, 20.7321)
  line L135 (-106.3397, 20.7321) -> (-110.6699, 23.2321)
  line L136 (-100.0096, 23.2321) -> (-104.3397, 20.7321)
  line L137 (-104.3397, 20.7321) -> (-104.3397, 15.7321)
  line L138 (-104.3397, 15.7321) -> (-100.0096, 13.2321)
  line L139 (-100.0096, 13.2321) -> (-95.6795, 15.7321)
  line L140 (-95.6795, 15.7321) -> (-95.6795, 20.7321)
  line L141 (-95.6795, 20.7321) -> (-100.0096, 23.2321)
  line L142 (-89.3494, 23.2321) -> (-93.6795, 20.7321)
  line L143 (-93.6795, 20.7321) -> (-93.6795, 15.7321)
  line L144 (-93.6795, 15.7321) -> (-89.3494, 13.2321)
  line L145 (-89.3494, 13.2321) -> (-85.0192, 15.7321)
  line L146 (-85.0192, 15.7321) -> (-85.0192, 20.7321)
  line L147 (-85.0192, 20.7321) -> (-89.3494, 23.2321)
  line L148 (-78.6891, 23.2321) -> (-83.0192, 20.7321)
  line L149 (-83.0192, 20.7321) -> (-83.0192, 15.7321)
  line L150 (-83.0192, 15.7321) -> (-78.6891, 13.2321)
  line L151 (-78.6891, 13.2321) -> (-74.359, 15.7321)
  line L152 (-74.359, 15.7321) -> (-74.359, 20.7321)
  line L153 (-74.359, 20.7321) -> (-78.6891, 23.2321)
  line L154 (-68.0289, 23.2321) -> (-72.359, 20.7321)
  line L155 (-72.359, 20.7321) -> (-72.359, 15.7321)
  line L156 (-72.359, 15.7321) -> (-68.0289, 13.2321)
  line L157 (-68.0289, 13.2321) -> (-63.6987, 15.7321)
  line L158 (-63.6987, 15.7321) -> (-63.6987, 20.7321)
  line L159 (-63.6987, 20.7321) -> (-68.0289, 23.2321)
  line L160 (-57.3686, 23.2321) -> (-61.6987, 20.7321)
  line L161 (-61.6987, 20.7321) -> (-61.6987, 15.7321)
  line L162 (-61.6987, 15.7321) -> (-57.3686, 13.2321)
  line L163 (-57.3686, 13.2321) -> (-53.0385, 15.7321)
  line L164 (-53.0385, 15.7321) -> (-53.0385, 20.7321)
  line L165 (-53.0385, 20.7321) -> (-57.3686, 23.2321)
  line L166 (-46.7083, 23.2321) -> (-51.0385, 20.7321)
  line L167 (-51.0385, 20.7321) -> (-51.0385, 15.7321)
  line L168 (-51.0385, 15.7321) -> (-46.7083, 13.2321)
  line L169 (-46.7083, 13.2321) -> (-42.3782, 15.7321)
  line L170 (-42.3782, 15.7321) -> (-42.3782, 20.7321)
  line L171 (-42.3782, 20.7321) -> (-46.7083, 23.2321)
  line L172 (-36.0481, 23.2321) -> (-40.3782, 20.7321)
  line L173 (-40.3782, 20.7321) -> (-40.3782, 15.7321)
  line L174 (-40.3782, 15.7321) -> (-36.0481, 13.2321)
  line L175 (-36.0481, 13.2321) -> (-31.718, 15.7321)
  line L176 (-31.718, 15.7321) -> (-31.718, 20.7321)
  line L177 (-31.718, 20.7321) -> (-36.0481, 23.2321)
  line L178 (-25.3878, 23.2321) -> (-29.718, 20.7321)
  line L179 (-29.718, 20.7321) -> (-29.718, 15.7321)
  line L180 (-29.718, 15.7321) -> (-25.3878, 13.2321)
  line L181 (-25.3878, 13.2321) -> (-21.0577, 15.7321)
  line L182 (-21.0577, 15.7321) -> (-21.0577, 20.7321)
  line L183 (-21.0577, 20.7321) -> (-25.3878, 23.2321)
  line L184 (-14.7276, 23.2321) -> (-19.0577, 20.7321)
  line L185 (-19.0577, 20.7321) -> (-19.0577, 15.7321)
  line L186 (-19.0577, 15.7321) -> (-14.7276, 13.2321)
  line L187 (-14.7276, 13.2321) -> (-10.3975, 15.7321)
  line L188 (-10.3975, 15.7321) -> (-10.3975, 20.7321)
  line L189 (-10.3975, 20.7321) -> (-14.7276, 23.2321)
  line L190 (-4.0673, 23.2321) -> (-8.3975, 20.7321)
  line L191 (-8.3975, 20.7321) -> (-8.3975, 15.7321)
  line L192 (-8.3975, 15.7321) -> (-4.0673, 13.2321)
  line L193 (-4.0673, 13.2321) -> (0.2628, 15.7321)
  line L194 (0.2628, 15.7321) -> (0.2628, 20.7321)
  line L195 (0.2628, 20.7321) -> (-4.0673, 23.2321)
  line L196 (6.5929, 23.2321) -> (2.2628, 20.7321)
  line L197 (2.2628, 20.7321) -> (2.2628, 15.7321)
  line L198 (2.2628, 15.7321) -> (6.5929, 13.2321)
  line L199 (6.5929, 13.2321) -> (10.923, 15.7321)
  line L200 (10.923, 15.7321) -> (10.923, 20.7321)
  line L201 (10.923, 20.7321) -> (6.5929, 23.2321)
  line L202 (17.2532, 23.2321) -> (12.923, 20.7321)
  line L203 (12.923, 20.7321) -> (12.923, 15.7321)
  line L204 (12.923, 15.7321) -> (17.2532, 13.2321)
  line L205 (17.2532, 13.2321) -> (21.5833, 15.7321)
  line L206 (21.5833, 15.7321) -> (21.5833, 20.7321)
  line L207 (21.5833, 20.7321) -> (17.2532, 23.2321)
  line L208 (27.9134, 23.2321) -> (23.5833, 20.7321)
  line L209 (23.5833, 20.7321) -> (23.5833, 15.7321)
  line L210 (23.5833, 15.7321) -> (27.9134, 13.2321)
  line L211 (27.9134, 13.2321) -> (32.2436, 15.7321)
  line L212 (32.2436, 15.7321) -> (32.2436, 20.7321)
  line L213 (32.2436, 20.7321) -> (27.9134, 23.2321)
  line L214 (38.5737, 23.2321) -> (34.2436, 20.7321)
  line L215 (34.2436, 20.7321) -> (34.2436, 15.7321)
  line L216 (34.2436, 15.7321) -> (38.5737, 13.2321)
  line L217 (38.5737, 13.2321) -> (42.9038, 15.7321)
  line L218 (42.9038, 15.7321) -> (42.9038, 20.7321)
  line L219 (42.9038, 20.7321) -> (38.5737, 23.2321)
  line L220 (49.2339, 23.2321) -> (44.9038, 20.7321)
  line L221 (44.9038, 20.7321) -> (44.9038, 15.7321)
  line L222 (44.9038, 15.7321) -> (49.2339, 13.2321)
  line L223 (49.2339, 13.2321) -> (53.5641, 15.7321)
  line L224 (53.5641, 15.7321) -> (53.5641, 20.7321)
  line L225 (53.5641, 20.7321) -> (49.2339, 23.2321)
  line L226 (59.8942, 23.2321) -> (55.5641, 20.7321)
  line L227 (55.5641, 20.7321) -> (55.5641, 15.7321)
  line L228 (55.5641, 15.7321) -> (59.8942, 13.2321)
  line L229 (59.8942, 13.2321) -> (64.2243, 15.7321)
  line L230 (64.2243, 15.7321) -> (64.2243, 20.7321)
  line L231 (64.2243, 20.7321) -> (59.8942, 23.2321)
  line L232 (70.5544, 23.2321) -> (66.2243, 20.7321)
  line L233 (66.2243, 20.7321) -> (66.2243, 15.7321)
  line L234 (66.2243, 15.7321) -> (70.5544, 13.2321)
  line L235 (70.5544, 13.2321) -> (74.8846, 15.7321)
  line L236 (74.8846, 15.7321) -> (74.8846, 20.7321)
  line L237 (74.8846, 20.7321) -> (70.5544, 23.2321)
  line L238 (81.2147, 23.2321) -> (76.8846, 20.7321)
  line L239 (76.8846, 20.7321) -> (76.8846, 15.7321)
  line L240 (76.8846, 15.7321) -> (81.2147, 13.2321)
  line L241 (81.2147, 13.2321) -> (85.5448, 15.7321)
  line L242 (85.5448, 15.7321) -> (85.5448, 20.7321)
  line L243 (85.5448, 20.7321) -> (81.2147, 23.2321)
  line L244 (91.875, 23.2321) -> (87.5448, 20.7321)
  line L245 (87.5448, 20.7321) -> (87.5448, 15.7321)
  line L246 (87.5448, 15.7321) -> (91.875, 13.2321)
  line L247 (91.875, 13.2321) -> (96.2051, 15.7321)
  line L248 (96.2051, 15.7321) -> (96.2051, 20.7321)
  line L249 (96.2051, 20.7321) -> (91.875, 23.2321)
  line L250 (102.5352, 23.2321) -> (98.2051, 20.7321)
  line L251 (98.2051, 20.7321) -> (98.2051, 15.7321)
  line L252 (98.2051, 15.7321) -> (102.5352, 13.2321)
  line L253 (102.5352, 13.2321) -> (106.8653, 15.7321)
  line L254 (106.8653, 15.7321) -> (106.8653, 20.7321)
  line L255 (106.8653, 20.7321) -> (102.5352, 23.2321)
  line L256 (-116, 32.4641) -> (-120.3301, 29.9641)
  line L257 (-120.3301, 29.9641) -> (-120.3301, 24.9641)
  line L258 (-120.3301, 24.9641) -> (-116, 22.4641)
  line L259 (-116, 22.4641) -> (-111.6699, 24.9641)
  line L260 (-111.6699, 24.9641) -> (-111.6699, 29.9641)
  line L261 (-111.6699, 29.9641) -> (-116, 32.4641)
  line L262 (-105.3397, 32.4641) -> (-109.6699, 29.9641)
  line L263 (-109.6699, 29.9641) -> (-109.6699, 24.9641)
  line L264 (-109.6699, 24.9641) -> (-105.3397, 22.4641)
  line L265 (-105.3397, 22.4641) -> (-101.0096, 24.9641)
  line L266 (-101.0096, 24.9641) -> (-101.0096, 29.9641)
  line L267 (-101.0096, 29.9641) -> (-105.3397, 32.4641)
  line L268 (-94.6795, 32.4641) -> (-99.0096, 29.9641)
  line L269 (-99.0096, 29.9641) -> (-99.0096, 24.9641)
  line L270 (-99.0096, 24.9641) -> (-94.6795, 22.4641)
  line L271 (-94.6795, 22.4641) -> (-90.3494, 24.9641)
  line L272 (-90.3494, 24.9641) -> (-90.3494, 29.9641)
  line L273 (-90.3494, 29.9641) -> (-94.6795, 32.4641)
  line L274 (-84.0192, 32.4641) -> (-88.3494, 29.9641)
  line L275 (-88.3494, 29.9641) -> (-88.3494, 24.9641)
  line L276 (-88.3494, 24.9641) -> (-84.0192, 22.4641)
  line L277 (-84.0192, 22.4641) -> (-79.6891, 24.9641)
  line L278 (-79.6891, 24.9641) -> (-79.6891, 29.9641)
  line L279 (-79.6891, 29.9641) -> (-84.0192, 32.4641)
  line L280 (-73.359, 32.4641) -> (-77.6891, 29.9641)
  line L281 (-77.6891, 29.9641) -> (-77.6891, 24.9641)
  line L282 (-77.6891, 24.9641) -> (-73.359, 22.4641)
  line L283 (-73.359, 22.4641) -> (-69.0289, 24.9641)
  line L284 (-69.0289, 24.9641) -> (-69.0289, 29.9641)
  line L285 (-69.0289, 29.9641) -> (-73.359, 32.4641)
  line L286 (-62.6987, 32.4641) -> (-67.0289, 29.9641)
  line L287 (-67.0289, 29.9641) -> (-67.0289, 24.9641)
  line L288 (-67.0289, 24.9641) -> (-62.6987, 22.4641)
  line L289 (-62.6987, 22.4641) -> (-58.3686, 24.9641)
  line L290 (-58.3686, 24.9641) -> (-58.3686, 29.9641)
  line L291 (-58.3686, 29.9641) -> (-62.6987, 32.4641)
  line L292 (-52.0385, 32.4641) -> (-56.3686, 29.9641)
  line L293 (-56.3686, 29.9641) -> (-56.3686, 24.9641)
  line L294 (-56.3686, 24.9641) -> (-52.0385, 22.4641)
  line L295 (-52.0385, 22.4641) -> (-47.7083, 24.9641)
  line L296 (-47.7083, 24.9641) -> (-47.7083, 29.9641)
  line L297 (-47.7083, 29.9641) -> (-52.0385, 32.4641)
  line L298 (-41.3782, 32.4641) -> (-45.7083, 29.9641)
  line L299 (-45.7083, 29.9641) -> (-45.7083, 24.9641)
  line L300 (-45.7083, 24.9641) -> (-41.3782, 22.4641)
  line L301 (-41.3782, 22.4641) -> (-37.0481, 24.9641)
  line L302 (-37.0481, 24.9641) -> (-37.0481, 29.9641)
  line L303 (-37.0481, 29.9641) -> (-41.3782, 32.4641)
  line L304 (-30.718, 32.4641) -> (-35.0481, 29.9641)
  line L305 (-35.0481, 29.9641) -> (-35.0481, 24.9641)
  line L306 (-35.0481, 24.9641) -> (-30.718, 22.4641)
  line L307 (-30.718, 22.4641) -> (-26.3878, 24.9641)
  line L308 (-26.3878, 24.9641) -> (-26.3878, 29.9641)
  line L309 (-26.3878, 29.9641) -> (-30.718, 32.4641)
  line L310 (-20.0577, 32.4641) -> (-24.3878, 29.9641)
  line L311 (-24.3878, 29.9641) -> (-24.3878, 24.9641)
  line L312 (-24.3878, 24.9641) -> (-20.0577, 22.4641)
  line L313 (-20.0577, 22.4641) -> (-15.7276, 24.9641)
  line L314 (-15.7276, 24.9641) -> (-15.7276, 29.9641)
  line L315 (-15.7276, 29.9641) -> (-20.0577, 32.4641)
  line L316 (-9.3975, 32.4641) -> (-13.7276, 29.9641)
  line L317 (-13.7276, 29.9641) -> (-13.7276, 24.9641)
  line L318 (-13.7276, 24.9641) -> (-9.3975, 22.4641)
  line L319 (-9.3975, 22.4641) -> (-5.0673, 24.9641)
  line L320 (-5.0673, 24.9641) -> (-5.0673, 29.9641)
  line L321 (-5.0673, 29.9641) -> (-9.3975, 32.4641)
  line L322 (1.2628, 32.4641) -> (-3.0673, 29.9641)
  line L323 (-3.0673, 29.9641) -> (-3.0673, 24.9641)
  line L324 (-3.0673, 24.9641) -> (1.2628, 22.4641)
  line L325 (1.2628, 22.4641) -> (5.5929, 24.9641)
  line L326 (5.5929, 24.9641) -> (5.5929, 29.9641)
  line L327 (5.5929, 29.9641) -> (1.2628, 32.4641)
  line L328 (11.923, 32.4641) -> (7.5929, 29.9641)
  line L329 (7.5929, 29.9641) -> (7.5929, 24.9641)
  line L330 (7.5929, 24.9641) -> (11.923, 22.4641)
  line L331 (11.923, 22.4641) -> (16.2532, 24.9641)
  line L332 (16.2532, 24.9641) -> (16.2532, 29.9641)
  line L333 (16.2532, 29.9641) -> (11.923, 32.4641)
  line L334 (22.5833, 32.4641) -> (18.2532, 29.9641)
  line L335 (18.2532, 29.9641) -> (18.2532, 24.9641)
  line L336 (18.2532, 24.9641) -> (22.5833, 22.4641)
  line L337 (22.5833, 22.4641) -> (26.9134, 24.9641)
  line L338 (26.9134, 24.9641) -> (26.9134, 29.9641)
  line L339 (26.9134, 29.9641) -> (22.5833, 32.4641)
  line L340 (33.2436, 32.4641) -> (28.9134, 29.9641)
  line L341 (28.9134, 29.9641) -> (28.9134, 24.9641)
  line L342 (28.9134, 24.9641) -> (33.2436, 22.4641)
  line L343 (33.2436, 22.4641) -> (37.5737, 24.9641)
  line L344 (37.5737, 24.9641) -> (37.5737, 29.9641)
  line L345 (37.5737, 29.9641) -> (33.2436, 32.4641)
  line L346 (43.9038, 32.4641) -> (39.5737, 29.9641)
  line L347 (39.5737, 29.9641) -> (39.5737, 24.9641)
  line L348 (39.5737, 24.9641) -> (43.9038, 22.4641)
  line L349 (43.9038, 22.4641) -> (48.2339, 24.9641)
  line L350 (48.2339, 24.9641) -> (48.2339, 29.9641)
  line L351 (48.2339, 29.9641) -> (43.9038, 32.4641)
  line L352 (54.5641, 32.4641) -> (50.2339, 29.9641)
  line L353 (50.2339, 29.9641) -> (50.2339, 24.9641)
  line L354 (50.2339, 24.9641) -> (54.5641, 22.4641)
  line L355 (54.5641, 22.4641) -> (58.8942, 24.9641)
  line L356 (58.8942, 24.9641) -> (58.8942, 29.9641)
  line L357 (58.8942, 29.9641) -> (54.5641, 32.4641)
  line L358 (65.2243, 32.4641) -> (60.8942, 29.9641)
  line L359 (60.8942, 29.9641) -> (60.8942, 24.9641)
  line L360 (60.8942, 24.9641) -> (65.2243, 22.4641)
  line L361 (65.2243, 22.4641) -> (69.5544, 24.9641)
  line L362 (69.5544, 24.9641) -> (69.5544, 29.9641)
  line L363 (69.5544, 29.9641) -> (65.2243, 32.4641)
  line L364 (75.8846, 32.4641) -> (71.5544, 29.9641)
  line L365 (71.5544, 29.9641) -> (71.5544, 24.9641)
  line L366 (71.5544, 24.9641) -> (75.8846, 22.4641)
  line L367 (75.8846, 22.4641) -> (80.2147, 24.9641)
  line L368 (80.2147, 24.9641) -> (80.2147, 29.9641)
  line L369 (80.2147, 29.9641) -> (75.8846, 32.4641)
  line L370 (86.5448, 32.4641) -> (82.2147, 29.9641)
  line L371 (82.2147, 29.9641) -> (82.2147, 24.9641)
  line L372 (82.2147, 24.9641) -> (86.5448, 22.4641)
  line L373 (86.5448, 22.4641) -> (90.875, 24.9641)
  line L374 (90.875, 24.9641) -> (90.875, 29.9641)
  line L375 (90.875, 29.9641) -> (86.5448, 32.4641)
  line L376 (97.2051, 32.4641) -> (92.875, 29.9641)
  line L377 (92.875, 29.9641) -> (92.875, 24.9641)
  line L378 (92.875, 24.9641) -> (97.2051, 22.4641)
  line L379 (97.2051, 22.4641) -> (101.5352, 24.9641)
  line L380 (101.5352, 24.9641) -> (101.5352, 29.9641)
  line L381 (101.5352, 29.9641) -> (97.2051, 32.4641)
  line L382 (-110.6699, 41.6962) -> (-115, 39.1962)
  line L383 (-115, 39.1962) -> (-115, 34.1962)
  line L384 (-115, 34.1962) -> (-110.6699, 31.6962)
  line L385 (-110.6699, 31.6962) -> (-106.3397, 34.1962)
  line L386 (-106.3397, 34.1962) -> (-106.3397, 39.1962)
  line L387 (-106.3397, 39.1962) -> (-110.6699, 41.6962)
  line L388 (-100.0096, 41.6962) -> (-104.3397, 39.1962)
  line L389 (-104.3397, 39.1962) -> (-104.3397, 34.1962)
  line L390 (-104.3397, 34.1962) -> (-100.0096, 31.6962)
  line L391 (-100.0096, 31.6962) -> (-95.6795, 34.1962)
  line L392 (-95.6795, 34.1962) -> (-95.6795, 39.1962)
  line L393 (-95.6795, 39.1962) -> (-100.0096, 41.6962)
  line L394 (-89.3494, 41.6962) -> (-93.6795, 39.1962)
  line L395 (-93.6795, 39.1962) -> (-93.6795, 34.1962)
  line L396 (-93.6795, 34.1962) -> (-89.3494, 31.6962)
  line L397 (-89.3494, 31.6962) -> (-85.0192, 34.1962)
  line L398 (-85.0192, 34.1962) -> (-85.0192, 39.1962)
  line L399 (-85.0192, 39.1962) -> (-89.3494, 41.6962)
  line L400 (-78.6891, 41.6962) -> (-83.0192, 39.1962)
  line L401 (-83.0192, 39.1962) -> (-83.0192, 34.1962)
  line L402 (-83.0192, 34.1962) -> (-78.6891, 31.6962)
  line L403 (-78.6891, 31.6962) -> (-74.359, 34.1962)
  line L404 (-74.359, 34.1962) -> (-74.359, 39.1962)
  line L405 (-74.359, 39.1962) -> (-78.6891, 41.6962)
  line L406 (-68.0289, 41.6962) -> (-72.359, 39.1962)
  line L407 (-72.359, 39.1962) -> (-72.359, 34.1962)
  line L408 (-72.359, 34.1962) -> (-68.0289, 31.6962)
  line L409 (-68.0289, 31.6962) -> (-63.6987, 34.1962)
  line L410 (-63.6987, 34.1962) -> (-63.6987, 39.1962)
  line L411 (-63.6987, 39.1962) -> (-68.0289, 41.6962)
  line L412 (-57.3686, 41.6962) -> (-61.6987, 39.1962)
  line L413 (-61.6987, 39.1962) -> (-61.6987, 34.1962)
  line L414 (-61.6987, 34.1962) -> (-57.3686, 31.6962)
  line L415 (-57.3686, 31.6962) -> (-53.0385, 34.1962)
  line L416 (-53.0385, 34.1962) -> (-53.0385, 39.1962)
  line L417 (-53.0385, 39.1962) -> (-57.3686, 41.6962)
  line L418 (-46.7083, 41.6962) -> (-51.0385, 39.1962)
  line L419 (-51.0385, 39.1962) -> (-51.0385, 34.1962)
  line L420 (-51.0385, 34.1962) -> (-46.7083, 31.6962)
  line L421 (-46.7083, 31.6962) -> (-42.3782, 34.1962)
  line L422 (-42.3782, 34.1962) -> (-42.3782, 39.1962)
  line L423 (-42.3782, 39.1962) -> (-46.7083, 41.6962)
  line L424 (-36.0481, 41.6962) -> (-40.3782, 39.1962)
  line L425 (-40.3782, 39.1962) -> (-40.3782, 34.1962)
  line L426 (-40.3782, 34.1962) -> (-36.0481, 31.6962)
  line L427 (-36.0481, 31.6962) -> (-31.718, 34.1962)
  line L428 (-31.718, 34.1962) -> (-31.718, 39.1962)
  line L429 (-31.718, 39.1962) -> (-36.0481, 41.6962)
  line L430 (-25.3878, 41.6962) -> (-29.718, 39.1962)
  line L431 (-29.718, 39.1962) -> (-29.718, 34.1962)
  line L432 (-29.718, 34.1962) -> (-25.3878, 31.6962)
  line L433 (-25.3878, 31.6962) -> (-21.0577, 34.1962)
  line L434 (-21.0577, 34.1962) -> (-21.0577, 39.1962)
  line L435 (-21.0577, 39.1962) -> (-25.3878, 41.6962)
  line L436 (-14.7276, 41.6962) -> (-19.0577, 39.1962)
  line L437 (-19.0577, 39.1962) -> (-19.0577, 34.1962)
  line L438 (-19.0577, 34.1962) -> (-14.7276, 31.6962)
  line L439 (-14.7276, 31.6962) -> (-10.3975, 34.1962)
  line L440 (-10.3975, 34.1962) -> (-10.3975, 39.1962)
  line L441 (-10.3975, 39.1962) -> (-14.7276, 41.6962)
  line L442 (-4.0673, 41.6962) -> (-8.3975, 39.1962)
  line L443 (-8.3975, 39.1962) -> (-8.3975, 34.1962)
  line L444 (-8.3975, 34.1962) -> (-4.0673, 31.6962)
  line L445 (-4.0673, 31.6962) -> (0.2628, 34.1962)
  line L446 (0.2628, 34.1962) -> (0.2628, 39.1962)
  line L447 (0.2628, 39.1962) -> (-4.0673, 41.6962)
  line L448 (6.5929, 41.6962) -> (2.2628, 39.1962)
  line L449 (2.2628, 39.1962) -> (2.2628, 34.1962)